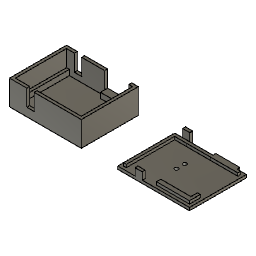
enclosure_v1 (Autodesk Fusion 360 design; units mm, degrees)
Autodesk Fusion 360 part; units mm, degrees
sketch "Sketch1" plane through (0, 0, 0) normal (0, 0, 1) x (1, 0, 0)
  line L0 (0, 0) -> (91.5, 0)
  line L1 (91.5, 0) -> (91.5, 71)
  line L2 (0, 0) -> (0, 71)
  line L3 (0, 71) -> (91.5, 71)
  line L4 (95.5, -4) -> (95.5, 75)
  line L5 (-4, 75) -> (95.5, 75)
  line L6 (-4, -4) -> (-4, 75)
  line L7 (-4, -4) -> (95.5, -4)
  line L8 (0, 0) -> (20, 0)
  line L9 (20, 0) -> (30, 0)
  line L10 (30, 0) -> (30, -4)
  line L11 (20, 0) -> (20, -4)
  line L12 (91.5, 71) -> (86.5, 71)
  line L13 (86.5, 71) -> (86.5, 75)
  line L14 (86.5, 71) -> (53, 71)
  line L15 (53, 71) -> (53, 75)
  line L16 (53, 71) -> (53, 65)
  line L17 (53, 65) -> (85, 65)
  line L18 (85, 65) -> (85, 6)
  line L19 (91.5, 0) -> (91.5, 6)
  line L20 (85, 6) -> (49.5, 6)
  line L21 (49.5, 6) -> (49.5, 0)
  line L22 (0, 0) -> (4, 0)
  line L23 (4, 0) -> (4, 71)
  line L24 (0, 71) -> (11, 71)
  line L25 (11, 71) -> (11, 75)
  line L26 (11, 71) -> (21, 71)
  line L27 (21, 71) -> (21, 75)
  line L28 (150, 71) -> (161, 71)
  line L29 (150, 0) -> (241.5, 0)
  line L30 (150, 71) -> (241.5, 71)
  line L31 (150, 0) -> (150, 71)
  line L32 (146, 75) -> (245.5, 75)
  line L33 (146, -4) -> (245.5, -4)
  line L34 (245.5, -4) -> (245.5, 75)
  line L35 (241.5, 0) -> (241.5, 6)
  line L36 (241.5, 0) -> (241.5, 71)
  line L37 (161, 71) -> (171, 71)
  line L38 (170, 0) -> (180, 0)
  line L39 (150, 0) -> (154, 0)
  line L40 (170, 0) -> (170, -4)
  line L41 (171, 71) -> (171, 75)
  line L42 (161, 71) -> (161, 75)
  line L43 (146, -4) -> (146, 75)
  line L44 (150, 0) -> (170, 0)
  line L45 (203, 71) -> (203, 75)
  line L46 (236.5, 71) -> (236.5, 75)
  line L47 (180, 0) -> (180, -4)
  line L48 (241.5, 71) -> (236.5, 71)
  line L49 (237.5, 6) -> (195.75, 6)
  line L50 (195.75, 6) -> (195.75, 0)
  line L51 (241.5, 0) -> (241.5, 15)
  line L52 (241.5, 15) -> (237.5, 15)
  line L53 (237.5, 15) -> (237.5, 6)
  line L54 (154, 0) -> (154, 71)
  line L55 (171, 67) -> (203, 67)
  line L56 (236.5, 67) -> (241.5, 67)
  line L57 (171, 67) -> (154, 67)
  line L58 (203, 67) -> (241.5, 67)
  circle A0 centre (190, 45) radius 2.5
  circle A1 centre (190, 33.5) radius 2.5
  dimension "d1" = 91.5
  dimension "d3" = 71
  dimension "d16" = 79
  dimension "d17" = 99.5
  dimension "d18" = 20
  dimension "d19" = 10
  dimension "d20" = 5
  dimension "d21" = 4
  dimension "d22" = 33.5
  dimension "d24" = 42
  dimension "d25" = 4
  dimension "d34" = 11
  dimension "d35" = 10
  dimension "d46" = 91.5
  dimension "d47" = 71
  dimension "d48" = 79
  dimension "d49" = 99.5
  dimension "d50" = 20
  dimension "d51" = 10
  dimension "d52" = 5
  dimension "d53" = 4
  dimension "d54" = 33.5
  dimension "d56" = 4
  dimension "d57" = 11
  dimension "d58" = 10
  dimension "d61" = 15
  dimension "d62" = 4
  dimension "d67" = 4
  dimension "d68" = 4
  dimension "d79" = 5
  dimension "d80" = 5
  constraint coincident L0.start L2.start
  constraint horizontal L0
  constraint perpendicular L0 L1
  constraint perpendicular L0 L2
  constraint horizontal L7
  constraint horizontal L5
  constraint vertical L6
  constraint coincident L4.start L7
  constraint perpendicular L4 L7
  constraint coincident L6 L7.start
  constraint coincident L4.end L5
  constraint perpendicular L2 L8
  constraint parallel L0 L9
  constraint coincident L7 L10.end
  constraint perpendicular L7 L10
  constraint perpendicular L8 L11
  constraint perpendicular L1 L12
  constraint perpendicular L12 L13
  constraint perpendicular L13 L14
  constraint coincident L5 L15.end
  constraint perpendicular L5 L15
  constraint perpendicular L3 L16
  constraint perpendicular L1 L17
  constraint perpendicular L0 L18
  constraint perpendicular L0 L19
  constraint perpendicular L19 L20
  constraint coincident L0 L21.end
  constraint perpendicular L0 L21
  constraint perpendicular L10 L22
  constraint coincident L3 L23.end
  constraint perpendicular L3 L23
  constraint perpendicular L2 L24
  constraint coincident L5 L25.end
  constraint perpendicular L5 L25
  constraint perpendicular L25 L26
  constraint coincident L5 L27.end
  constraint perpendicular L5 L27
  constraint horizontal L29
  constraint perpendicular L29 L36
  constraint perpendicular L29 L31
  constraint horizontal L33
  constraint horizontal L32
  constraint vertical L43
  constraint coincident L34.start L33
  constraint perpendicular L33 L34
  constraint coincident L33.start L43
  constraint coincident L34.end L32
  constraint perpendicular L31 L44
  constraint parallel L29 L38
  constraint coincident L47.end L33
  constraint perpendicular L33 L47
  constraint perpendicular L40 L44
  constraint perpendicular L36 L48
  constraint perpendicular L46 L48
  constraint coincident L45.end L32
  constraint perpendicular L32 L45
  constraint perpendicular L29 L35
  constraint perpendicular L39 L47
  constraint perpendicular L28 L31
  constraint coincident L42.end L32
  constraint perpendicular L32 L42
  constraint perpendicular L37 L42
  constraint coincident L41.end L32
  constraint perpendicular L32 L41
  constraint perpendicular L36 L49
  constraint midpoint L29 L50.end
  constraint perpendicular L29 L50
  constraint perpendicular L29 L51
  constraint perpendicular L36 L52
  constraint perpendicular L49 L53
  constraint coincident L28 L54.end
  constraint coincident L30 L54.end
  constraint coincident L36 L56.end
  constraint perpendicular L36 L56
  constraint coincident L54 L57.end
  constraint perpendicular L54 L57
  measures "d1" distance of L0.start L0.end
  measures "d3" distance of L0.start L2.end
  measures "d16" distance of L4.end L4.start
  measures "d17" distance of L4.end L5.start
  measures "d18" distance of L0.start L8.end
  measures "d19" distance of L8.end L9.end
  measures "d20" distance of L1.end L12.end
  measures "d21" distance of L12.end L13.end
  measures "d22" distance of L12.end L14.end
  measures "d24" distance of L19.end L20.end
  measures "d25" distance of L0.start L22.end
  measures "d34" distance of L2.end L24.end
  measures "d35" distance of L24.end L26.end
  measures "d46" distance of L29.end L29.start
  measures "d47" distance of L29.start L28.start
  measures "d48" distance of L33.end L32.end
  measures "d49" distance of L32.start L32.end
  measures "d50" distance of L29.start L38.start
  measures "d51" distance of L38.start L38.end
  measures "d52" distance of L46.start L30.end
  measures "d53" distance of L46.start L46.end
  measures "d54" distance of L45.start L46.start
  measures "d56" distance of L39.end L29.start
  measures "d57" distance of L28.end L28.start
  measures "d58" distance of L37.end L28.end
  measures "d61" distance of L29.end L51.end
  measures "d62" distance of L51.end L52.end
  measures "d67" distance of L37.end L55.start
  measures "d68" distance of L45.start L55.end
  measures "d79" diameter of A0
  measures "d80" diameter of A1
extrude "Extrude1" add sketch "Sketch1" along normal blind 7.5 contours L0 L1 L3 L12 L14 L16 L17 L18 L19 L20 L21 makes body 1
extrude "Extrude2" add sketch "Sketch1" along normal blind 7.5 separate body contours L0 L2 L3 L8 L22 L23 L24 makes body 2
extrude "Extrude3" add sketch "Sketch1" along normal blind 7.5 separate body contours L0 L7 L9 L10 L11 makes body 3
extrude "Extrude4" add sketch "Sketch1" along normal blind 7.5 contours L3 L5 L13 L14 L15 bodies 1
extrude "Extrude5" add sketch "Sketch1" along normal blind 30.5 contours L0 L1 L3 L4 L5 L7 L10 L12 L13 L19 bodies 1 3
extrude "Extrude6" add sketch "Sketch1" along normal blind 30.5 contours L3 L5 L15 L27 bodies 1
extrude "Extrude7" add sketch "Sketch1" along normal blind 7.5 contours L3 L5 L25 L26 L27 bodies 1
extrude "Extrude8" add sketch "Sketch1" along normal blind 30.5 contours L0 L2 L3 L5 L6 L7 L8 L11 L22 L24 L25 bodies 1 2
extrude "Extrude9" add sketch "Sketch1" against normal blind 4 separate body contours L0 L2 L3 L8 L22 L23 L24 | L0 L2 L3 L5 L6 L7 L8 L11 L22 L24 L25 | L0 L3 L8 L9 L16 L17 L18 L20 L21 L23 L24 L26 | L0 L7 L9 L10 L11 | L0 L1 L3 L4 L5 L7 L10 L12 L13 L19 | L3 L5 L25 L26 L27 | L0 L1 L3 L12 L14 L16 L17 L18 L19 L20 L21 | L3 L5 L15 L27 | L3 L5 L13 L14 L15 makes body 4
combine "Combine1" operation add target body 1 tool bodies 4
extrude "Extrude10" add sketch "Sketch1" against normal blind 4 separate body contours L28 L29 L30 L31 L32 L33 L39 L40 L42 L43 L44 | L28 L29 L30 L31 L39 L44 L54 | L28 L30 L36 L37 L48 L54 L55 L56 L57 L58 | L30 L32 L37 L41 L42 | L29 L36 L38 L44 L49 L50 L52 L53 L54 L55 L56 L57 L58 | L30 L32 L41 L45 | L29 L33 L38 L40 L47 | L30 L32 L45 L46 | L29 L30 L32 L33 L34 L35 L36 L46 L47 L48 L51 | L29 L35 L36 L49 L50 L51 L52 L53 | A0 | A1 makes body 5
extrude "Extrude11" add sketch "Sketch1" along normal blind 4 contours L28 L29 L30 L31 L39 L44 L54 bodies 5
extrude "Extrude12" add sketch "Sketch1" along normal blind 4 contours L29 L35 L36 L49 L50 L51 L52 L53 bodies 5
extrude "Extrude13" add sketch "Sketch1" along normal blind 4 contours L28 L30 L36 L37 L48 L54 L55 L56 L57 L58 bodies 5
extrude "Extrude14" add sketch "Sketch1" along normal blind 4 contours L28 L30 L36 L37 L48 L54 L55 L56 L57 L58 bodies 5
extrude "Extrude15" add sketch "Sketch1" along normal blind 10 contours L29 L33 L38 L40 L47 bodies 5
extrude "Extrude16" add sketch "Sketch1" along normal blind 15 separate body contours L30 L32 L37 L41 L42 makes body 6
extrude "Extrude17" add sketch "Sketch1" along normal blind 4 contours L30 L32 L45 L46 bodies 5
extrude "Extrude18" cut sketch "Sketch1" against normal blind 10 contours A0 | A1 bodies 5
combine "Combine2" operation add target body 6 tool bodies 5
named bodies: "bottom", "top"
